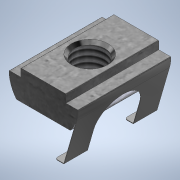
# Autodesk Inventor part: NUT, SPRING, MK, M8
Saved by Autodesk Inventor 2022.3 (Build 263350000, 350)
## iProperties
Created: 2012-03-26
Material: Steel, MS
Document SubType Name: Modeling
Designer: robr , Rob
Manufacturer: Standard
Standards Organization: Custom
Density: 7.86 g/cm^3
Checked By: 21N1M
Engr Approved By: R
User Status: Work In Process
Description: NUT, SPRING, MK, M8
Mfg Approved By: Rob.Roddy
Appearance: Steel Galvanized
Part Number: NUT, SPRING, MK, M8
Mass: 11.059 g
Surface Area: 12.705 cm^2
Volume: 1.407 cm^3
Manager: 100-29256
Category: _
CN_SERVICEABLE: _
FIRST_DESCRIPTION: NUT, SPRING, MK, M8
PTC_WM_ITERATION: 5
PTC_WM_ORGANIZATION_ID: CLWC
PTC_WM_LIFECYCLE: CLWC_CAD_LC
CN_MASS: 0.01105898341340876
CL_runCount: 1
FinishProperty: ToBeSet
SECOND_DESCRIPTION: _
THIRD_DESCRIPTION: _
Author: -
Subject: 34.16.0831
Revision Number: 1
Keywords: -
Autodesk Inventor part; units mm, degrees
ref_plane "YZ Plane" through (0, 0, 0) normal (1, 0, 0) x (0, 1, 0)
ref_plane "XZ Plane" through (0, 0, 0) normal (0, 1, 0) x (-1, 0, 0)
ref_plane "XY Plane" through (0, 0, 0) normal (0, 0, 1) x (1, 0, 0)
sketch "Sketch1" plane through (0, 0, 0) normal (0, 0, 1) x (1, 0, 0)
  line L0 (-4.8895, 1.7272) -> (4.8895, 1.7272)
  line L1 (4.8895, 1.7272) -> (4.8895, 0)
  line L2 (4.8895, 0) -> (7.4295, 0)
  line L3 (-4.8895, 1.7272) -> (-4.8895, 0)
  line L4 (-4.8895, 0) -> (-7.4295, 0)
  line L5 (0, 1.7272) -> (0, -4.6228) construction
  line L6 (-5.8161, -4.6228) -> (5.8161, -4.6228)
  arc A0 (5.8161, -4.6228) -> (7.4295, 0) centre (0, 0) ccw
  arc A1 (-7.4295, 0) -> (-5.8161, -4.6228) centre (0, 0) ccw
  dimension "d0" = 14.859
  dimension "d1" = 9.779
  dimension "d2" = 1.7272
  dimension "d3" = 6.35
  constraints: 14 end point, 5 perpendicular, 4 point on circle, 3 midpoint, 2 centre point, 2 coincident, 2 collinear, 2 point on line, 1 horizontal, 1 parallel
  measures "d0" distance of L4.end L2.end
  measures "d1" distance between parallel lines of L3 L1
  measures "d2" distance between parallel lines of L2 L0
  measures "d3" distance between parallel lines of L0 L6
extrude "Extrusion1" add sketch "Sketch1" along normal mid plane 20
sketch "Sketch2" plane through (-4.8895, 1.7272, 10) normal (0, 1, 0) x (1, 0, 0)
  point P0 (4.8895, 10)
  point P1 (4.8895, 10)
  constraints: 1 coincident
hole "Hole1" at (0, 1.7272, 0) direction (0, -1, 0) diameter 6.647 end through all thread size "M8x1.25" class "6H" standard "ANSI Metric M Profile"
sketch "Sketch3" plane through (0, 0, 0) normal (0, 0, 1) x (1, 0, 0)
  line L0 (2.54, -11.4938) -> (4.321, -11.4938)
  arc A0 (4.321, -11.4938) -> (4.4305, -11.4115) centre (4.321, -11.3798) ccw
  line L1 (4.4305, -11.4115) -> (7.1364, -2.0663)
  line L2 (7.2459, -2.098) -> (4.54, -11.4432)
  arc A1 (4.321, -11.6078) -> (4.54, -11.4432) centre (4.321, -11.3798) ccw
  line L3 (4.321, -11.6078) -> (2.54, -11.6078)
  line L4 (2.54, -11.6078) -> (2.54, -11.4938)
  arc A2 (7.2459, -2.098) -> (7.5435, 0) centre (0, 0) ccw
  line L5 (7.4295, 0) -> (7.5435, 0)
  arc A3 (7.1364, -2.0663) -> (7.4295, 0) centre (0, 0) ccw
  line L6 (7.4295, 0) -> (4.8895, 0) projected
  line L7 (4.8895, 1.7272) -> (-4.8895, 1.7272) projected
  dimension "d16" = 0.114
  dimension "d17" = 0.114
  dimension "d18" = 2
  dimension "d20" = 13.335
  dimension "d21" = 2.54
  constraints: 12 end point, 8 point on circle, 6 tangent, 4 centre point, 2 coincident, 2 parallel, 2 perpendicular, 1 collinear
  measures "d16" radius of A0
  measures "d17" distance between parallel lines of L3 L0
  measures "d18" distance from line of L4 L2.end
  measures "d20" distance between parallel lines of L7 L3
  measures "d21" distance from line of A2.centre L4
extrude "Extrusion2" add sketch "Sketch3" along normal mid plane 20
sketch "Sketch4" plane through (7.1364, -2.0663, -10) normal (-0.9605462, 0.2781205, 0) x (0, 0, 1)
  line L0 (10, 0) -> (10, 0)
  line L1 (15, -5) -> (15, -10.4434)
  line L2 (15, -10.4434) -> (5, -10.4434)
  line L3 (5, -10.4434) -> (5, -5)
  line L4 (20, -10.4434) -> (0, -10.4434) projected
  arc A0 (15, -5) -> (10, 0) centre (10, -5) ccw
  arc A1 (10, 0) -> (5, -5) centre (10, -5) ccw
  line L5 (20, 0) -> (0, 0) projected
  point P0 (10, 0)
  point P1 (10, -10.4434)
  dimension "d24" = 10
  dimension "d25" = 5
  constraints: 8 end point, 5 tangent, 4 point on circle, 2 centre point, 2 midpoint, 2 parallel, 1 concentric, 1 horizontal, 1 perpendicular, 1 point on line
  measures "d24" distance between parallel lines of L3 L1
  measures "d25" radius of A0
extrude "Extrusion3" cut sketch "Sketch4" against normal through all
sketch "Sketch5" plane through (7.2459, -2.098, 10) normal (0.9605462, -0.2781205, 0) x (0, 0, -1)
  line L0 (5, -5) -> (15, -5)
  line L1 (15, -5) -> (15, -10.4434)
  line L2 (15, -10.4434) -> (5, -10.4434)
  line L3 (5, -10.4434) -> (5, -5)
  line L4 (0, -10.4434) -> (20, -10.4434) projected
  line L5 (15, -5) -> (15, -9.7291) projected
  constraints: 8 end point, 2 parallel, 2 point on line, 1 horizontal, 1 perpendicular
extrude "Extrusion4" cut sketch "Sketch5" against normal blind 3
fillet "Fillet1" radius 0.5 4 edges at (2.54, -11.5508, 10) (2.54, -11.5508, 5) (2.54, -11.5508, -5) (2.54, -11.5508, -10)
fillet "Fillet2" radius 0.125 6 edges at (4.8895, 1.7272, 0) (-4.8895, 1.7272, 0) (-7.4295, 0, 0) (5.8161, -4.6228, 0) (-5.8161, -4.6228, 0) (7.5435, 0, 0)
chamfer "Chamfer1" distance 0.625 angle 45 2 edges at (0, 1.7272, -3.3235) (0, -4.6228, -3.3235)
equation "\"d16\" = d17"
body "Solid1"
